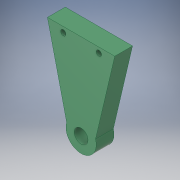
# Autodesk Inventor part: joint3_rot
Saved by Autodesk Inventor 2019 (Build 230136000, 136)
## iProperties
Created: 2019-12-29
Part Number: joint3_rot
Material: Пластик АБС
Document SubType Name: Modeling
Designer: Петров Иван
Density: 1.06 g/cm^3
Appearance: Гладкий — темный цвет морской волны
Author: Петров Иван
Autodesk Inventor part; units mm, degrees
ref_plane "YZ Plane" through (0, 0, 0) normal (1, 0, 0) x (0, 1, 0)
ref_plane "XZ Plane" through (0, 0, 0) normal (0, 1, 0) x (-1, 0, 0)
ref_plane "XY Plane" through (0, 0, 0) normal (0, 0, 1) x (1, 0, 0)
sketch "Эскиз1" plane through (0, 0, 0) normal (0, 0, 1) x (1, 0, 0)
  circle A0 centre (0, 0) radius 3.9
  line L0 (-3.9, 0) -> (-3.9, 42.320681)
  line L1 (3.9, 42.320681) -> (3.9, 0)
  arc A1 (3.9, 42.320681) -> (-3.9, 42.320681) centre (0, 0) ccw
  line L2 (-3.9, 42.320681) -> (-3.9, 48.320681)
  line L3 (-3.9, 48.320681) -> (3.9, 48.320681)
  line L4 (3.9, 48.320681) -> (3.9, 42.320681)
  circle A2 centre (0, 0) radius 7.5
  point P0 (0, 0)
  point P1 (0, -39)
  dimension "d0" = 0
  dimension "d1" = 6
  dimension "d2" = 15
  constraints: 10 end point, 4 point on circle, 3 centre point, 2 perpendicular, 2 vertical, 1 coincident, 1 parallel, 1 tangent
  measures "d0" distance of A0.centre A1.centre
  measures "d1" distance of L0.end L2.end
  measures "d2" diameter of A2
extrude "Выдавливание1" add sketch "Эскиз1" along normal blind 10 contours L1 A2 L0 A0 | A0 L0 A2 L1 | A2 L0 A1 L1 | A1 L2 L3 L4
sketch "Эскиз3" plane through (0, 0, 10) normal (0, 0, 1) x (1, 0, 0)
  line L0 (3.9, 48.320681) -> (-3.9, 48.320681)
  line L1 (-3.9, 48.320681) -> (-18.9, 48.320681)
  line L2 (-18.9, 48.320681) -> (-7.5, 0)
  arc A0 (-3.9, 6.406247) -> (3.9, 6.406247) centre (0, 0) ccw
  line L3 (3.9, 6.406247) -> (3.9, 48.320681)
  line L4 (3.9, 48.320681) -> (18.9, 48.320681)
  line L5 (18.9, 48.320681) -> (7.5, 0)
  arc A1 (7.5, 0) -> (-7.5, 0) centre (0, 0) ccw
  line L6 (-3.9, 48.320681) -> (-3.9, 43.72824)
  line L7 (-3.9, 43.72824) -> (3.9, 43.72824)
  line L8 (3.9, 48.320681) -> (3.9, 43.72824)
  point P0 (0, 0)
  dimension "d13" = 15
  dimension "d14" = 15
  constraints: 14 end point, 4 point on circle, 2 horizontal, 1 centre point, 1 collinear, 1 concentric, 1 perpendicular, 1 point on line, 1 vertical
  measures "d13" distance of L0.end L1.end
  measures "d14" distance of L0.start L4.end
extrude "Выдавливание3" add sketch "Эскиз3" against normal blind 10 contours L4 L5 A0 L3 | L6 L7 L3 A1 A0 L2 L1
sketch "Эскиз4" plane through (0, 0, 10) normal (0, 0, 1) x (1, 0, 0)
  line L0 (18.9, 48.320681) -> (-18.9, 48.320681)
  line L1 (0, 48.320681) -> (0, 45.320681)
  line L2 (0, 45.320681) -> (-10, 45.320681)
  line L3 (-10, 45.320681) -> (10, 45.320681)
  circle A0 centre (-10, 45.320681) radius 1.5
  circle A1 centre (10, 45.320681) radius 1.5
  point P0 (0, 0)
  dimension "d17" = 3
  dimension "d18" = 10
  dimension "d19" = 20
  dimension "d20" = 3
  dimension "d21" = 3
  constraints: 6 end point, 2 centre point, 2 coincident, 1 midpoint, 1 perpendicular, 1 point on line, 1 vertical
  measures "d17" distance of L1.start L1.end
  measures "d18" distance of L1.end L2.end
  measures "d19" distance of L2.end L3.end
  measures "d20" diameter of A0
  measures "d21" diameter of A1
extrude "Выдавливание4" cut sketch "Эскиз4" against normal blind 10
thicken "Толщина2" operation add thickness 1 both sides no extend neighbours yes toward (-0.9870503, -0.1604113, 0) faces at (-7.402877, -1.203085, 3.333333)
equation "\"d14\" = d13"
